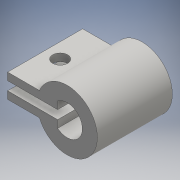
# Autodesk Inventor part: DShaftClamp
Saved by Autodesk Inventor 2016 (Build 200138000, 138)
## iProperties
Created: 2017-11-27
Part Number: DShaftClamp
Material: Generic
Document SubType Name: Modeling
Designer: alex
Density: 1 g/cm^3
Appearance: Default
Author: alex
Autodesk Inventor part; units mm, degrees
ref_plane "YZ Plane" through (0, 0, 0) normal (1, 0, 0) x (0, 1, 0)
ref_plane "XZ Plane" through (0, 0, 0) normal (0, 1, 0) x (-1, 0, 0)
ref_plane "XY Plane" through (0, 0, 0) normal (0, 0, 1) x (1, 0, 0)
sketch "Sketch1" plane through (0, 0, 0) normal (0, 1, 0) x (-1, 0, 0)
  arc A0 (5.5375, 2.3691) -> (5.5375, -2.3691) centre (-0.0185, 0) ccw
  arc A1 (1.8865, 2.3691) -> (1.8865, -2.3691) centre (-0.0185, 0) ccw
  line L0 (5.5375, -2.3691) -> (11.8865, -2.3691)
  line L1 (11.8865, -2.3691) -> (11.8865, -0.8691)
  line L2 (11.8865, -0.8691) -> (1.8865, -0.8691)
  line L3 (1.8865, -0.8691) -> (1.8865, -2.3691)
  line L4 (5.5375, 2.3691) -> (11.8865, 2.3691)
  line L5 (11.8865, 2.3691) -> (11.8865, 0.8691)
  line L6 (11.8865, 0.8691) -> (1.8865, 0.8691)
  line L7 (1.8865, 0.8691) -> (1.8865, 2.3691)
  point P0 (11.8865, -1.6191)
  point P1 (11.8865, 1.6191)
  dimension "d146" = 6.08
  dimension "d147" = 3
  dimension "d151" = 1.5
  dimension "d152" = 10
  dimension "d158" = 10
  dimension "d159" = 1.7382
  dimension "d160" = 3.2382
  dimension "d161" = 6.349
  dimension "d162" = 6.349
  constraints: 16 end point, 4 parallel, 4 point on circle, 2 centre point, 2 horizontal, 2 midpoint, 2 perpendicular, 1 coincident, 1 vertical alignment
  measures "d146" diameter of A1
  measures "d147" radial gap between concentric circles of A0 A1
  measures "d151" distance of L4.end L5.end
  measures "d152" distance of L1.end L2.end
  measures "d158" distance between parallel lines of L7 L5
  measures "d159" distance between parallel lines of L6 L2
  measures "d160" distance between parallel lines of L0 L6
  measures "d161" distance from line of L4.start L5
  measures "d162" distance from line of L0.start L5
extrude "Extrusion3" add sketch "Sketch1" along normal blind 15
sketch "Sketch3" plane through (-5.5375, 0, -2.3691) normal (0, 0, -1) x (-1, 0, 0)
  circle A0 centre (3.349, 7.5) radius 1.5
  line L0 (0, 15) -> (6.349, 15) projected
  line L1 (0, 0) -> (6.349, 0) projected
  line L2 (6.349, 0) -> (6.349, 15) projected
  point P0 (-5.5375, 0)
  point P1 (6.349, 7.5)
  dimension "d165" = 3
  dimension "d169" = 3
  constraints: 1 centre point, 1 horizontal alignment, 1 midpoint
  measures "d165" diameter of A0
  measures "d169" distance from line of L2 A0.centre
extrude "Extrusion5" cut sketch "Sketch3" against normal through all
body "Solid2"
